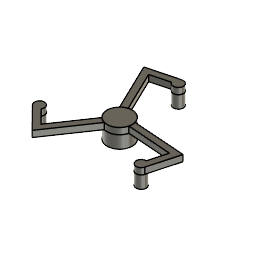
bearing rotor v2 (Autodesk Fusion 360 design; units mm, degrees)
part number: 2026-04-22-23-42-39-207
Autodesk Fusion 360 part; units mm, degrees
sketch "Sketch1" plane through (0, 0, 0) normal (0, 0, 1) x (1, 0, 0)
  circle A0 centre (0, 0) radius 31.75 construction
  line L0 (0, 27.546) -> (0, -31.973) construction
  line L1 (-40.4824, 0) -> (36.5438, 0) construction
  line L2 (0, 1.75) -> (0, 22.5)
  line L3 (1.75, 0) -> (22.5, 0)
  line L4 (-2, 1.5) -> (2, 1.5)
  line L5 (-2, -1.5) -> (2, -1.5)
  circle A1 centre (0, 0) radius 5.08
  arc A2 (-2, 1.5) -> (-2, -1.5) centre (0, 0) ccw
  arc A3 (2, -1.5) -> (2, 1.5) centre (0, 0) ccw
  circle A4 centre (0, 23.726) radius 6.5 construction
  circle A5 centre (0, 23.726) radius 2.05
  line L6 (7.62, 30.226) -> (-7.158, 30.226) construction
  line L7 (-11.43, 31.75) -> (19.6746, 31.75) construction
  dimension "d1" = 63.5
  dimension "d3" = 5
  dimension "d4" = 3
  dimension "d5" = 10.16
  dimension "d6" = 2.5
  dimension "d7" = 13
  dimension "d8" = 4.1
  dimension "d18" = 1.524
  constraint coincident A0.centre A1.centre
  constraint vertical L0
  constraint horizontal L1
  constraint collinear L0 L2
  constraint collinear L1 L3
  constraint concentric A0 A2
  constraint perpendicular L0 L4
  constraint perpendicular L0 L5
  constraint symmetric L1 L4 L5
  constraint concentric A0 A1
  constraint concentric A2 A3
  constraint coincident L0 A4.centre
  constraint concentric A4 A5
  constraint horizontal L6
  constraint horizontal L7
  constraint tangent A4 L6
  constraint tangent A0 L7
  measures "d1" diameter of A0
  measures "d3" diameter of A2
  measures "d4" distance of L4 L5
  measures "d5" diameter of A1
  measures "d6" radius of A3
  measures "d7" diameter of A4
  measures "d8" diameter of A5
  measures "d18" distance of L6 L7
extrude "Extrude1" add sketch "Sketch1" along normal blind 5.08 makes body 1 at (2.0398, 23.5219, 1.6933) makes body 2 at (5.0548, -0.5058, 1.6933)
sketch "Sketch2" plane through (0, 0, 5.08) normal (0, 0, 1) x (-1, 0, 0)
  arc A0 (2, -1.5) -> (2, 1.5) centre (0, 0) ccw
  line L0 (2, -1.5) -> (-2, -1.5)
  arc A1 (-2, 1.5) -> (-2, -1.5) centre (0, 0) ccw
  line L1 (-2, 1.5) -> (2, 1.5)
  circle A2 centre (0, 0) radius 5.08
  line L2 (0.5814, -25.6929) -> (12.7461, -22.5093)
  line L3 (12.7461, -22.5093) -> (2.9238, -2.1591)
  line L4 (-0.0617, -23.2356) -> (9.1169, -20.8335)
  line L5 (9.1169, -20.8335) -> (0.6363, -3.2632)
  line L6 (2.9238, -2.1591) -> (0.6363, -3.2632)
  line L7 (0.5814, -25.6929) -> (-0.0617, -23.2356)
  circle A3 centre (0, -23.726) radius 2.05
  dimension "d21" = 90
  dimension "d26" = 2.54
  dimension "d27" = 2.54
  constraint parallel L3 L5
  constraint parallel L2 L4
  constraint perpendicular L4 L7
  constraint tangent L2 A3
  measures "d21" angle of L3 L6
  measures "d26" distance of L2 L4
  measures "d27" distance of L3 L5
extrude "Extrude3" add sketch "Sketch2" 1 faces at (0.4261, 24.4639, 5.08) along normal blind 2.54 separate body contours A0 L0 A1 L1 | A2 L3 L5 L6 | A2 L3 L5 L6 | A2 L2 L3 L4 L5 A3 | L4 L7 A3 picked at (0.4581, -24.8393) on bodies 1 makes body 3
pattern_circular "C-Pattern3" count 3 over 360 about axis through (0, 0, 1.75) along (0, 0, 1) of bodies 3 1 makes body 4 at (-21.744, -10.1985, 3.3867) makes body 5 at (19.7042, -13.7316, 3.3867) makes body 6 at (-9.2992, -15.1727, 5.08) makes body 7 at (17.7895, -0.4671, 5.08)
